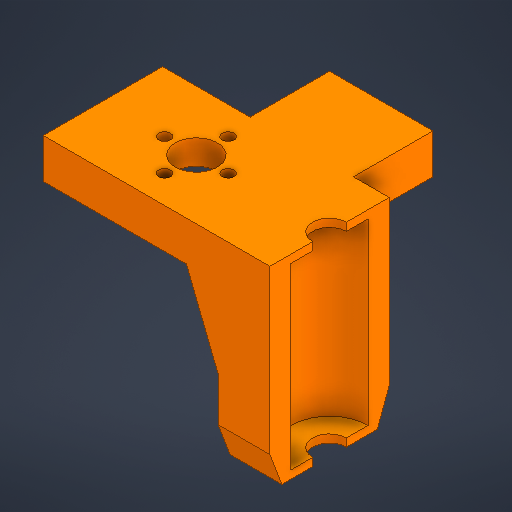
# Autodesk Inventor part: Z axis bracket
Saved by Autodesk Inventor 2025.1 (Build 291241000, 241)
## iProperties
Created: 2024-11-11
Part Number: Z axis bracket
Material: Generic
Document SubType Name: Modeling
Designer: jerem
Density: 1 g/cm^3
Appearance: Default
Author: jerem
Autodesk Inventor part; units mm, degrees
ref_plane "YZ Plane" through (0, 0, 0) normal (1, 0, 0) x (0, 1, 0)
ref_plane "XZ Plane" through (0, 0, 0) normal (0, 1, 0) x (-1, 0, 0)
ref_plane "XY Plane" through (0, 0, 0) normal (0, 0, 1) x (1, 0, 0)
sketch "Sketch1" plane through (0, 0, 0) normal (0, 1, 0) x (-1, 0, 0)
  circle A0 centre (0, 0) radius 7.7
  circle A1 centre (0, 0) radius 9.7
  line L0 (0, 0) -> (33.5, 0) construction
  circle A2 centre (33.5, 0) radius 4.25 construction
  circle A3 centre (0, 0) radius 4.25
  circle A4 centre (33.5, 0) radius 5.3
  circle A5 centre (33.5, 0) radius 11.25
  circle A6 centre (41.5, 0) radius 1.5
  line L1 (41.5, 0) -> (33.5, 0) construction
  line L2 (57, 15) -> (-13, 15)
  line L3 (-13, 15) -> (-13, -15)
  line L4 (-13, -15) -> (57, -15)
  line L5 (57, -15) -> (57, 15)
  line L6 (0, 0) -> (-13, 0) construction
  line L7 (32, -15) -> (32, -35)
  line L8 (12, -35) -> (12, -15)
  line L9 (22, -35) -> (22, -15) construction
  line L10 (32, -35) -> (22, -35)
  line L11 (12, -35) -> (22, -35)
  line L12 (32, -35) -> (35, -35)
  line L13 (35, -35) -> (35, -15)
  line L14 (12, -35) -> (9, -35)
  line L15 (9, -35) -> (9, -15)
  circle A7 centre (33.5, 8) radius 1.5
  circle A8 centre (25.5, 0) radius 1.5
  circle A9 centre (33.5, -8) radius 1.5
  line L16 (13, 15) -> (13, -15)
  line L17 (0, 15) -> (0, -15)
  point P0 (0, 9.7)
  point P1 (0, -9.7)
  point P2 (0, 4.25)
  point P3 (0, -4.25)
  point P4 (0, 7.7)
  point P5 (0, -7.7)
  dimension "d0" = 15.4
  dimension "d1" = 2
  dimension "d2" = 33.5
  dimension "d3" = 8.5
  dimension "d4" = 8.5
  dimension "d5" = 10.6
  dimension "d6" = 22.5
  dimension "d7" = 3
  dimension "d8" = 8
  dimension "d9" = 70
  dimension "d10" = 20
  dimension "d11" = 30
  dimension "d13" = 3
  dimension "d14" = 20
  dimension "d19" = 360
  dimension "d23" = 13
  dimension "d24" = 13
  constraints: 34 end point, 10 centre point, 7 vertical, 6 horizontal, 5 coincident, 3 collinear, 3 point on line, 2 midpoint, 2 perpendicular, 1 parallel, 19 other
  measures "d0" diameter of A0
  measures "d1" radial gap between concentric circles of A0 A1
  measures "d2" distance of L0.start L0.end
  measures "d3" diameter of A3
  measures "d4" diameter of A2
  measures "d5" diameter of A4
  measures "d6" diameter of A5
  measures "d7" diameter of A6
  measures "d8" distance of L1.start L1.end
  measures "d9" distance of L2.start L2.end
  measures "d10" distance between parallel lines of L7 L8
  measures "d11" distance of L2.end L3.end
  measures "d13" distance between parallel lines of L7 L13
  measures "d23" distance from line of L16 L0.start
  measures "d24" distance from line of L0.start L3
extrude "Extrusion1" add sketch "Sketch1" along normal blind 10 contours L2 L5 L4 L16 | L4 L8 L14 L15 | L4 L7 L10 L11 L8 | L4 L13 L12 L7 | A5
extrude "Extrusion2" cut sketch "Sketch1" along normal blind 3.8 from surface at 0 contours A5
extrude "Extrusion3" add sketch "Sketch1" along normal blind 8 and the other way blind 37 contours L17 L2 L16 L4 A1
extrude "Extrusion4" add sketch "Sketch1" along normal blind 2 from surface at 8 contours A0 L17 A3 | A0 L17 A1 | L17 L2 L16 L4 A1 picked at (6.4501, -0.8864) picked at (8.8879, -1.2906)
extrude "Extrusion6" add sketch "Sketch1" against normal blind 2 from surface at -37 contours A0 L17 A3 | A0 L17 A1 | L17 L2 L16 L4 A1 picked at (6.4501, -0.8864) picked at (8.8879, -1.2906)
chamfer "Chamfer1" distance 3 distance2 8 2 edges at (-6.5, -39, 15) (-6.5, -39, -15) measured on face at (-6.5, -39, 14.5) measured on face at (-6.5, -39, -14.5)
chamfer "Chamfer2" distance 8 distance2 20 1 edges at (-13, 0, 0) measured on face at (-13.5, 0, 0)
equation "\"d24\" = d23"
equation "\"d27\" = d1"
body "Solid1"
